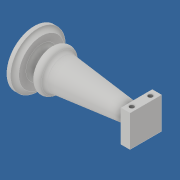
# Autodesk Inventor part: Maschienensäule
Saved by Autodesk Inventor 2018 (Build 220112000, 112)
## iProperties
Created: 2018-09-18
Part Number: Maschienensäule
Material: Generisch
Document SubType Name: Modeling
Designer: M.Knabel
Density: 1 g/cm^3
Appearance: Vorgabe
Author: M.Knabel
Autodesk Inventor part; units mm, degrees
ref_plane "YZ Plane" through (0, 0, 0) normal (1, 0, 0) x (0, 1, 0)
ref_plane "XZ Plane" through (0, 0, 0) normal (0, 1, 0) x (-1, 0, 0)
ref_plane "XY Plane" through (0, 0, 0) normal (0, 0, 1) x (1, 0, 0)
sketch "Skizze1" plane through (0, 0, 0) normal (0, 0, 1) x (1, 0, 0)
  line L0 (-11.1647, 0) -> (66.9884, 0) projected
  line L1 (0, -2.95) -> (0, 17.7) projected
  line L2 (0, 14.75) -> (0, 0)
  line L3 (0, 14.75) -> (2, 14.75)
  arc A0 (2, 14.75) -> (4, 12.25) centre (4.5625, 14.75) ccw
  line L4 (4, 12.25) -> (4, 8.5)
  arc A1 (4, 8.5) -> (9, 8.5) centre (6.5, 8.5) ccw
  arc A2 (50.8907, 4.8) -> (55, 8.5) centre (51.2796, 8.5) ccw
  line L5 (55, 8.5) -> (55, 0)
  line L6 (0, 0) -> (55, 0)
  arc A3 (50.8907, 4.8) -> (55, 8.5) centre (51.2796, 8.5) ccw
  line L7 (19.0176, 8.15) -> (50.8907, 4.8)
  arc A4 (4, 8.5) -> (9, 8.5) centre (6.5, 8.5) ccw
  arc A5 (13.6654, 9.7494) -> (9, 8.5) centre (11.5, 8.5) ccw
  line L8 (50.8907, 4.8) -> (15.5695, 8.5124)
  arc A6 (13.6654, 9.7494) -> (15.5695, 8.5124) centre (15.8309, 10.9987) ccw
  dimension "d0" = 29.5
  dimension "d1" = 24.5
  dimension "d2" = 4
  dimension "d3" = 2
  dimension "d7" = 12
  dimension "d10" = 9.6
  dimension "d11" = 9
  dimension "d12" = 17
  dimension "d13" = 55
  dimension "d18" = 6
  dimension "d20" = 16.3
  dimension "d24" = 22
  dimension "d25" = 6
  dimension "d26" = 2.5
  constraints: 14 end point, 14 point on circle, 7 centre point, 7 tangent, 3 point on line, 2 coincident, 2 collinear, 2 horizontal alignment, 1 concentric, 1 horizontal, 1 perpendicular, 1 vertical
  measures "d0" diameter of L3 L0
  measures "d1" diameter of L4.start L0
  measures "d2" distance between parallel lines of L2 L4
  measures "d3" distance from line of L2 L3.end
  measures "d10" diameter of L7.end L0
  measures "d11" distance from line of A1.end L1
  measures "d12" diameter of L5.start L0
  measures "d13" distance between parallel lines of L1 L5
  measures "d18" angle of L6 L7
  measures "d20" diameter of L7.start L0
  measures "d25" angle of L0 L8
  measures "d26" radius of A6
revolve "Grundkörper dre" add sketch "Skizze1" angle 360 about axis through (-10, 0, 0) along (1, 0, 0)
sketch "Skizze2" plane through (55, 0, 0) normal (1, 0, 0) x (0, 0, -1)
  circle A0 centre (0, 0) radius 12.25 projected
  line L0 (20.65, 0) -> (-20.65, 0) projected
  line L1 (0, -20.65) -> (0, 20.65) projected
  line L2 (-8.5, 8.5) -> (8.5, 8.5)
  line L3 (8.5, 8.5) -> (8.5, -8.5)
  circle A1 centre (0, 0) radius 11 projected
  line L4 (-8.5, 8.5) -> (-8.5, -8.5)
  line L5 (-8.5, -8.5) -> (8.5, -8.5)
  circle A2 centre (0, 0) radius 8.5 projected
  point P0 (8.5, 0)
  dimension "d31" = 17
  dimension "d32" = 17
  constraints: 8 end point, 1 horizontal, 1 horizontal alignment, 1 midpoint, 1 perpendicular, 1 vertical, 2 other
  measures "d31" distance between parallel lines of L3 L4
  measures "d32" distance between parallel lines of L5 L2
extrude "Grundkörper ex" add sketch "Skizze2" along normal blind 5 contours A2 L1 L0 | A2 L2 A1 L3 | L0 L1 A2 | L3 A1 L5 A2 | A1 L2 L3 | L3 L5 A1 | A2 L4 A1 L2 | L1 L0 A2 | A1 L4 L2 | A2 L0 L1 | L5 A1 L4 A2 | L5 L4 A1
sketch "Skizze3" plane through (55, -8.5, 8.5) normal (0, 0, 1) x (1, 0, 0)
  line L0 (-67, 8.5) -> (17, 8.5) projected
  line L1 (0, 0) -> (0, 8.5) projected
  line L2 (0, 0) -> (5, 0) projected
  line L3 (5, 17) -> (5, 0) projected
  line L4 (0, 17) -> (5, 17) projected
  line L5 (0, 8.5) -> (0, 17) projected
  point P0 (-55, 8.5)
  point P1 (2.5, 3.5)
  point P2 (2.5, 13.5)
  dimension "d35" = 2.5
  dimension "d36" = 2.5
  dimension "d37" = 10
  constraints: 1 symmetric about line, 1 vertical alignment
  measures "d35" distance from line of L1 point (2.5, 3.5)
  measures "d36" distance from line of L5 point (2.5, 13.5)
  measures "d37" distance of point (2.5, 13.5) point (2.5, 3.5)
hole "Bohrung1" at (57.5, -5, 8.5) at (57.5, 5, 8.5) direction (0, 0, -1) diameter 2.459 end through all thread size "M3x0.5" class "6H" standard "ISO Metric profile"
sketch "Skizze4" plane through (0, 0, 0) normal (-1, 0, 0) x (0, 0, 1)
  point P0 (0, 0)
  point P1 (0, 0)
  constraints: 1 coincident
hole "Bohrung2" at (0, 0, 0) direction (1, 0, 0) diameter 3.242 depth 10 tip angle 118 thread size "M4x0.7" class "6H" standard "ISO Metric profile"
